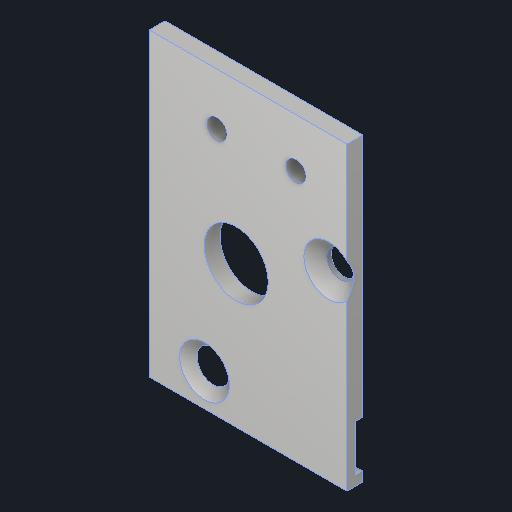
# Autodesk Inventor part: OslonaPrawejPrzekladni
Saved by Autodesk Inventor 2023 (Build 270158000, 158)
## iProperties
Created: 2022-03-19
Part Number: OslonaPrawejPrzekladni
Material: Aluminium 6061
Document SubType Name: Modeling
Designer: Michał
Density: 2.7 g/cm^3
Appearance: Aluminium — płaski
Mass: 0.679318 g
Surface Area: 4.32522 cm^2
Volume: 0.251599 cm^3
Author: Michał
Autodesk Inventor part; units mm, degrees
ref_plane "YZ Plane" through (0, 0, 0) normal (1, 0, 0) x (0, 1, 0)
ref_plane "XZ Plane" through (0, 0, 0) normal (0, 1, 0) x (-1, 0, 0)
ref_plane "XY Plane" through (0, 0, 0) normal (0, 0, 1) x (1, 0, 0)
sketch "Szkic1" plane through (0, 0, 0) normal (0, 0, 1) x (1, 0, 0)
  line L0 (12.5, 18.6) -> (12.5, -19.4) projected
  line L1 (-12.5, 18.6) -> (12.5, 18.6) projected
  line L2 (12.5, -19.4) -> (-12.5, -19.4)
  line L3 (-12.5, -19.4) -> (-12.5, 18.6)
  line L4 (-12.5, 18.6) -> (12.5, 18.6)
  line L5 (12.5, 18.6) -> (12.5, -19.4)
  constraints: 8 end point, 2 parallel, 1 horizontal, 1 perpendicular
extrude "Wyciągnięcie proste1" add sketch "Szkic1" along normal blind 2
sketch "Szkic2" plane through (0, 0, 2) normal (0, 0, 1) x (1, 0, 0)
  circle A0 centre (-3.9514, 12.0297) radius 1.25 projected
  circle A1 centre (6.0405, 12.4305) radius 1.25 projected
  circle A2 centre (-1.5, -1.5) radius 4.05 projected
  circle A3 centre (10.2, 3.6) radius 1.2295 projected
  point P0 (0, 0)
  point P1 (-5.5, -15.25)
  constraints: 1 coincident, 1 other
extrude "Wyciągnięcie proste2" cut sketch "Szkic2" against normal through all contours A0 | A1 | A2
hole "Otwór1" at (10.2, 3.6, 2) at (-5.5, -15.25, 2) direction (0, 0, -1) diameter 3.4 depth 7 tip angle 118 countersink diameter 6.3 countersink angle 90 clearance for "Śruba ze łbem stożkowym ISO 2009/7046" size "M3" standard "ISO"
sketch "Szkic3" plane through (12.5, -18.6, 0) normal (1, 0, 0) x (0, 0, -1)
  line L0 (0, 0.4) -> (-0.9, 0.4)
  line L1 (-0.9, 0.4) -> (-0.9, 6.3)
  line L2 (-0.9, 6.3) -> (0, 6.3)
  line L3 (0, 6.3) -> (0, 0.4)
  point P0 (0, 18.6)
  dimension "d11" = 0.9
  constraints: 8 end point, 2 parallel, 1 coincident, 1 horizontal, 1 perpendicular, 2 other
  measures "d11" distance of L1.end L2.end
extrude "Wyciągnięcie proste3" cut sketch "Szkic3" against normal blind 23
